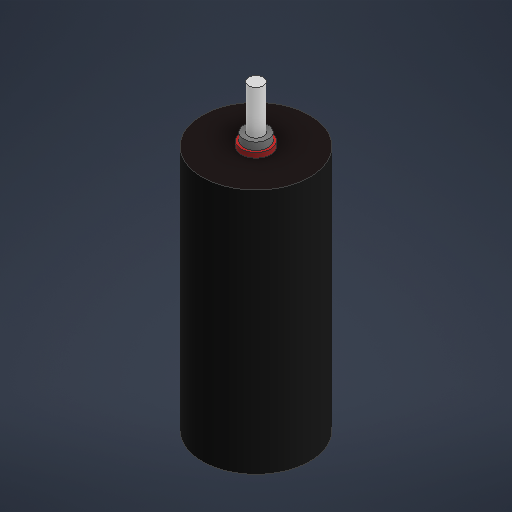
# Autodesk Inventor part: MotorStanger
Saved by Autodesk Inventor 2026.1 (Build 301233000, 233)
## iProperties
Created: 2025-10-13
Part Number: MotorStanger
Material: Generisch
Document SubType Name: Modeling
Designer: JurijLenz
Density: 1 g/cm^3
Appearance: Vorgabe
Author: JurijLenz
Autodesk Inventor part; units mm, degrees
ref_plane "YZ Plane" through (0, 0, 0) normal (1, 0, 0) x (0, 1, 0)
ref_plane "XZ Plane" through (0, 0, 0) normal (0, 1, 0) x (-1, 0, 0)
ref_plane "XY Plane" through (0, 0, 0) normal (0, 0, 1) x (1, 0, 0)
sketch "Skizze1" plane through (0, 0, 0) normal (0, 0, 1) x (1, 0, 0)
  circle A0 centre (0, 0) radius 11
  dimension "d0" = 22
  constraints: 1 centre point, 1 coincident
  measures "d0" diameter of A0
extrude "Extrusion1" add sketch "Skizze1" along normal blind 50.5
sketch "Skizze2" plane through (0, 0, 50.5) normal (0, 0, 1) x (1, 0, 0)
  circle A0 centre (0, 0) radius 3
  circle A1 centre (0, 0) radius 2.5
  circle A2 centre (0, 0) radius 1.5
  dimension "d3" = 6
  dimension "d4" = 5
  dimension "d9" = 3
  constraints: 3 centre point, 3 coincident
  measures "d3" diameter of A0
  measures "d4" diameter of A1
  measures "d9" diameter of A2
extrude "Extrusion2" add sketch "Skizze2" along normal blind 1 contours A0 | A1 | A2
extrude "Extrusion3" add sketch "Skizze2" along normal blind 2.5 contours A1 | A2
extrude "Extrusion4" add sketch "Skizze2" along normal blind 11.5 contours A2
